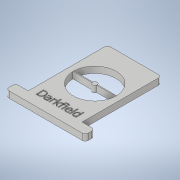
# Autodesk Inventor part: 00_Slider_Mask_Darkfield
Saved by Autodesk Inventor 2022 (Build 260153000, 153)
## iProperties
Created: 2021-10-22
Part Number: 00_Slider_Mask_Darkfield
Material: Generic
Document SubType Name: Modeling
Designer: diederichbenedict
Density: 1 g/cm^3
Appearance: Default
Author: diederichbenedict
Autodesk Inventor part; units mm, degrees
ref_plane "YZ Plane" through (0, 0, 0) normal (1, 0, 0) x (0, 1, 0)
ref_plane "XZ Plane" through (0, 0, 0) normal (0, 1, 0) x (-1, 0, 0)
ref_plane "XY Plane" through (0, 0, 0) normal (0, 0, 1) x (1, 0, 0)
sketch "Sketch1" plane through (0, 0, 0) normal (0, 1, 0) x (-1, 0, 0)
  line L0 (-17, 25) -> (17, 25)
  line L1 (17, 25) -> (17, -25)
  line L2 (17, -25) -> (-17, -25)
  line L3 (-17, -25) -> (-17, 25)
  line L4 (-17, 25) -> (17, -25) construction
  line L5 (17, 25) -> (-17, -25) construction
  line L6 (9, -17) -> (9, 17)
  line L7 (9, 17) -> (-9, 17)
  line L8 (-9, 17) -> (-9, -17)
  line L9 (-9, -17) -> (9, -17)
  line L10 (-25, 31) -> (25, 31)
  line L11 (25, 31) -> (25, 25)
  line L12 (25, 25) -> (-25, 25)
  line L13 (-25, 25) -> (-25, 31)
  line L14 (-25, 31) -> (25, 25) construction
  line L15 (25, 31) -> (-25, 25) construction
  point P0 (0, 0)
  point P1 (0, 28)
  point P2 (0, 25)
  dimension "d0" = 34
  dimension "d1" = 50
  dimension "d2" = 8
  dimension "d3" = 50
  dimension "d4" = 6
  constraints: 32 end point, 6 midpoint, 6 parallel, 3 perpendicular, 2 horizontal, 3 other
  measures "d0" distance of L1.end L2.end
  measures "d1" distance of L0.end L1.end
  measures "d2" distance between parallel lines of L1 L6
  measures "d3" distance of L11.end L12.end
  measures "d4" distance of L10.end L11.end
extrude "Extrusion1" add sketch "Sketch1" along normal blind 4 contours L12 L13 L10 L11 L0 | L0 L1 L2 L3 | L9 L8 L7 L6
sketch "Sketch2" plane through (0, 4, 0) normal (0, 1, 0) x (1, 0, 0)
  line L0 (25, -25) -> (17, -25)
  line L1 (17, -25) -> (17, 25)
  line L2 (17, 25) -> (-17, 25)
  line L3 (-17, 25) -> (-17, -25)
  line L4 (-17, -25) -> (-25, -25)
  line L5 (-25, -25) -> (-25, -31)
  line L6 (-25, -31) -> (25, -31)
  line L7 (25, -31) -> (25, -25)
  line L8 (13.5, 17) -> (-13.5, 17)
  line L9 (-13.5, 17) -> (-13.5, -17)
  line L10 (-13.5, -17) -> (13.5, -17)
  line L11 (13.5, -17) -> (13.5, 17)
  line L12 (13.5, 17) -> (-13.5, -17) construction
  line L13 (-13.5, 17) -> (13.5, -17) construction
  circle A0 centre (0, 0) radius 13.5
  circle A1 centre (0, 0) radius 1.5
  line L14 (-1.469694, 0.3) -> (-13.999729, 0.3)
  line L15 (-13.999729, 0.3) -> (-13.999729, -0.3)
  line L16 (-13.999729, -0.3) -> (-1.469694, -0.3)
  line L17 (-1.469694, -0.3) -> (-1.469694, 0.3)
  line L18 (1.469694, 0.3) -> (13.971759, 0.3)
  line L19 (13.971759, 0.3) -> (13.971759, -0.3)
  line L20 (13.971759, -0.3) -> (1.469694, -0.3)
  line L21 (1.469694, -0.3) -> (1.469694, 0.3)
  point P0 (13.496666, -0.3)
  point P1 (13.5, -0.3)
  point P2 (13.5, 0)
  point P3 (13.5, 0.3)
  point P4 (13.496666, 0.3)
  point P5 (1.469694, -0.3)
  point P6 (1.469694, -0.3)
  point P7 (-1.469694, -0.3)
  point P8 (-1.469694, -0.3)
  point P9 (-13.496666, -0.3)
  point P10 (-13.5, -0.3)
  point P11 (-13.5, 0)
  point P12 (-13.496666, 0.3)
  point P13 (-13.5, 0.3)
  dimension "d7" = 27
  dimension "d8" = 34
  dimension "d14" = 0.3
  dimension "d15" = 0.3
  dimension "d16" = 3
  constraints: 28 end point, 6 parallel, 3 horizontal, 3 perpendicular, 2 centre point, 2 coincident, 2 midpoint, 2 point on circle, 2 point on line
  measures "d7" distance of L10.end L9.end
  measures "d8" distance of L9.end L8.end
  measures "d14" distance from line of point (0, 0) L14
  measures "d15" distance from line of point (0, 0) L16
  measures "d16" diameter of A1
sketch "Sketch2 outline for Extrusion2" plane through (0, 4, 0) normal (0, 1, 0) x (1, 0, 0)
  line L0 (13.496666, -0.3) -> (13.5, -0.3)
  arc A0 (13.5, 0) -> (13.496666, -0.3) centre (0, 0) cw
  line L1 (13.5, -0.3) -> (13.5, 0)
  line L2 (13.5, 0.3) -> (13.496666, 0.3)
  line L3 (13.5, 0) -> (13.5, 0.3)
  arc A1 (13.496666, 0.3) -> (13.5, 0) centre (0, 0) cw
  line L4 (13.496666, -0.3) -> (1.469694, -0.3)
  arc A2 (-13.496666, -0.3) -> (13.496666, -0.3) centre (0, 0) ccw
  line L5 (-1.469694, -0.3) -> (-13.496666, -0.3)
  arc A3 (1.469694, -0.3) -> (-1.469694, -0.3) centre (0, 0) cw
  line L6 (-1.469694, -0.3) -> (-1.469694, 0.3)
  arc A4 (-1.469694, 0.3) -> (-1.469694, -0.3) centre (0, 0) ccw
  line L7 (-13.5, -0.3) -> (-13.496666, -0.3)
  line L8 (-13.5, 0) -> (-13.5, -0.3)
  arc A5 (-13.496666, -0.3) -> (-13.5, 0) centre (0, 0) cw
  line L9 (1.469694, 0.3) -> (1.469694, -0.3)
  arc A6 (1.469694, -0.3) -> (1.469694, 0.3) centre (0, 0) ccw
  line L10 (-13.496666, 0.3) -> (-13.5, 0.3)
  arc A7 (-13.5, 0) -> (-13.496666, 0.3) centre (0, 0) cw
  line L11 (-13.5, 0.3) -> (-13.5, 0)
  line L12 (1.469694, 0.3) -> (13.496666, 0.3)
  arc A8 (-1.469694, 0.3) -> (1.469694, 0.3) centre (0, 0) cw
  line L13 (-13.496666, 0.3) -> (-1.469694, 0.3)
  arc A9 (13.496666, 0.3) -> (-13.496666, 0.3) centre (0, 0) ccw
extrude "Extrusion2" cut sketch "Sketch2 outline for Extrusion2" against normal through all contours A0 L1 L0 | A2 L5 A3 L4 | A1 L2 L3 | L9 A6 | L7 L8 A5 | L12 A8 L13 A9 | A4 L6 | L11 L10 A7
sketch "Sketch3" plane through (0, 4, 0) normal (0, 1, 0) x (1, 0, 0)
  line L0 (-13.184715, -19.253856) -> (12.041103, -19.253856) construction
  line L1 (12.041103, -19.253856) -> (12.041103, -24.441026) construction
  line L2 (12.041103, -24.441026) -> (-13.184715, -24.441026) construction
  line L3 (-13.184715, -24.441026) -> (-13.184715, -19.253856) construction
  spline S0 degree 2 poles (-8.853526, -21.94014) (-8.853526, -22.60678) (-9.393939, -23.679716) (-9.84757, -23.979506) knots 0 0 0 1 2 2 2
  spline S1 degree 2 poles (-9.84757, -23.979506) (-10.218364, -24.212239) (-10.979674, -24.370023) (-11.571367, -24.370023) knots 0 0 0 1 2 2 2
  line L4 (-11.571367, -24.370023) -> (-12.691638, -24.370023)
  line L5 (-12.691638, -24.370023) -> (-12.691638, -19.502367)
  line L6 (-12.691638, -19.502367) -> (-11.583201, -19.502367)
  spline S2 degree 2 poles (-11.583201, -19.502367) (-10.896837, -19.502367) (-10.115804, -19.707487) (-9.83968, -19.88894) knots 0 0 0 1 2 2 2
  spline S3 degree 2 poles (-9.83968, -19.88894) (-9.370271, -20.200564) (-8.853526, -21.230109) (-8.853526, -21.94014) knots 0 0 0 1 2 2 2
  spline S4 degree 2 poles (-9.528056, -21.932251) (-9.528056, -21.372115) (-9.89885, -20.579248) (-10.265699, -20.354404) knots 0 0 0 1 2 2 2
  spline S5 degree 2 poles (-10.265699, -20.354404) (-10.526044, -20.200564) (-11.113791, -20.062503) (-11.551644, -20.062503) knots 0 0 0 1 2 2 2
  line L7 (-11.551644, -20.062503) -> (-12.044721, -20.062503)
  line L8 (-12.044721, -20.062503) -> (-12.044721, -23.809888)
  line L9 (-12.044721, -23.809888) -> (-11.551644, -23.809888)
  spline S6 degree 2 poles (-11.551644, -23.809888) (-11.121681, -23.809888) (-10.470819, -23.671826) (-10.20653, -23.486429) knots 0 0 0 1 2 2 2
  spline S7 degree 2 poles (-10.20653, -23.486429) (-9.867293, -23.257642) (-9.528056, -22.500275) (-9.528056, -21.932251) knots 0 0 0 1 2 2 2
  spline S8 degree 2 poles (-6.163298, -23.983451) (-6.238246, -24.038676) (-6.490702, -24.235906) (-6.60904, -24.295076) knots 0 0 0 1 2 2 2
  spline S9 degree 2 poles (-6.60904, -24.295076) (-6.770769, -24.381857) (-7.074505, -24.472583) (-7.350628, -24.472583) knots 0 0 0 1 2 2 2
  spline S10 degree 2 poles (-7.350628, -24.472583) (-7.575471, -24.472583) (-7.981766, -24.302965) (-8.135606, -24.149125) knots 0 0 0 1 2 2 2
  spline S11 degree 2 poles (-8.135606, -24.149125) (-8.281557, -23.999229) (-8.459065, -23.557432) (-8.459065, -23.312866) knots 0 0 0 1 2 2 2
  spline S12 degree 2 poles (-8.459065, -23.312866) (-8.459065, -22.934183) (-8.139551, -22.397715) (-7.792425, -22.243875) knots 0 0 0 1 2 2 2
  spline S13 degree 2 poles (-7.792425, -22.243875) (-7.484745, -22.101869) (-6.648486, -21.995365) (-6.163298, -21.967752) knots 0 0 0 1 2 2 2
  line L10 (-6.163298, -21.967752) -> (-6.163298, -21.849414)
  spline S14 degree 2 poles (-6.163298, -21.849414) (-6.163298, -21.636405) (-6.293471, -21.372115) (-6.411809, -21.297168) knots 0 0 0 1 2 2 2
  spline S15 degree 2 poles (-6.411809, -21.297168) (-6.530148, -21.22222) (-6.869385, -21.174885) (-7.050837, -21.174885) knots 0 0 0 1 2 2 2
  spline S16 degree 2 poles (-7.050837, -21.174885) (-7.263846, -21.174885) (-7.83976, -21.301112) (-8.127717, -21.423395) knots 0 0 0 1 2 2 2
  line L11 (-8.127717, -21.423395) -> (-8.163219, -21.423395)
  line L12 (-8.163219, -21.423395) -> (-8.163219, -20.796201)
  spline S17 degree 2 poles (-8.163219, -20.796201) (-7.9936, -20.748866) (-7.358517, -20.630528) (-7.046892, -20.630528) knots 0 0 0 1 2 2 2
  spline S18 degree 2 poles (-7.046892, -20.630528) (-6.668209, -20.630528) (-6.151465, -20.748866) (-5.946345, -20.902706) knots 0 0 0 1 2 2 2
  spline S19 degree 2 poles (-5.946345, -20.902706) (-5.745169, -21.052601) (-5.547938, -21.5299) (-5.547938, -21.873082) knots 0 0 0 1 2 2 2
  line L13 (-5.547938, -21.873082) -> (-5.547938, -24.370023)
  line L14 (-5.547938, -24.370023) -> (-6.163298, -24.370023)
  line L15 (-6.163298, -24.370023) -> (-6.163298, -23.983451)
  line L16 (-6.163298, -23.470651) -> (-6.163298, -22.456885)
  spline S20 degree 2 poles (-6.163298, -22.456885) (-6.384197, -22.476608) (-7.050837, -22.543666) (-7.259902, -22.60678) knots 0 0 0 1 2 2 2
  spline S21 degree 2 poles (-7.259902, -22.60678) (-7.504468, -22.681728) (-7.823982, -22.993352) (-7.823982, -23.269476) knots 0 0 0 1 2 2 2
  spline S22 degree 2 poles (-7.823982, -23.269476) (-7.823982, -23.585045) (-7.468966, -23.904559) (-7.129729, -23.904559) knots 0 0 0 1 2 2 2
  spline S23 degree 2 poles (-7.129729, -23.904559) (-6.841772, -23.904559) (-6.368418, -23.656048) (-6.163298, -23.470651) knots 0 0 0 1 2 2 2
  line L17 (-2.747261, -21.37606) -> (-2.778818, -21.37606)
  spline S24 degree 2 poles (-2.778818, -21.37606) (-2.849821, -21.356337) (-3.003661, -21.348448) (-3.110166, -21.348448) knots 0 0 0 1 2 2 2
  spline S25 degree 2 poles (-3.110166, -21.348448) (-3.358677, -21.348448) (-3.847809, -21.565401) (-4.068707, -21.778411) knots 0 0 0 1 2 2 2
  line L18 (-4.068707, -21.778411) -> (-4.068707, -24.370023)
  line L19 (-4.068707, -24.370023) -> (-4.684068, -24.370023)
  line L20 (-4.684068, -24.370023) -> (-4.684068, -20.717309)
  line L21 (-4.684068, -20.717309) -> (-4.068707, -20.717309)
  line L22 (-4.068707, -20.717309) -> (-4.068707, -21.261666)
  spline S26 degree 2 poles (-4.068707, -21.261666) (-3.733415, -20.961875) (-3.232449, -20.717309) (-2.995772, -20.717309) knots 0 0 0 1 2 2 2
  spline S27 degree 2 poles (-2.995772, -20.717309) (-2.901101, -20.717309) (-2.80643, -20.725198) (-2.747261, -20.737032) knots 0 0 0 1 2 2 2
  line L23 (-2.747261, -20.737032) -> (-2.747261, -21.37606)
  line L24 (0.755558, -24.370023) -> (-0.053089, -24.370023)
  line L25 (-0.053089, -24.370023) -> (-1.410036, -22.60678)
  line L26 (-1.410036, -22.60678) -> (-1.654603, -22.843457)
  line L27 (-1.654603, -22.843457) -> (-1.654603, -24.370023)
  line L28 (-1.654603, -24.370023) -> (-2.269963, -24.370023)
  line L29 (-2.269963, -24.370023) -> (-2.269963, -19.285414)
  line L30 (-2.269963, -19.285414) -> (-1.654603, -19.285414)
  line L31 (-1.654603, -19.285414) -> (-1.654603, -22.259654)
  line L32 (-1.654603, -22.259654) -> (-0.210873, -20.717309)
  line L33 (-0.210873, -20.717309) -> (0.554382, -20.717309)
  line L34 (0.554382, -20.717309) -> (-0.944572, -22.243875)
  line L35 (-0.944572, -22.243875) -> (0.755558, -24.370023)
  line L36 (2.984266, -19.877106) -> (2.952709, -19.877106)
  spline S28 degree 2 poles (2.952709, -19.877106) (2.869872, -19.845549) (2.562192, -19.790324) (2.439909, -19.790324) knots 0 0 0 1 2 2 2
  spline S29 degree 2 poles (2.439909, -19.790324) (2.053336, -19.790324) (1.721989, -20.137451) (1.721989, -20.595026) knots 0 0 0 1 2 2 2
  line L37 (1.721989, -20.595026) -> (1.721989, -20.717309)
  line L38 (1.721989, -20.717309) -> (2.739699, -20.717309)
  line L39 (2.739699, -20.717309) -> (2.739699, -21.226165)
  line L40 (2.739699, -21.226165) -> (1.741712, -21.226165)
  line L41 (1.741712, -21.226165) -> (1.741712, -24.370023)
  line L42 (1.741712, -24.370023) -> (1.126352, -24.370023)
  line L43 (1.126352, -24.370023) -> (1.126352, -21.226165)
  line L44 (1.126352, -21.226165) -> (0.712167, -21.226165)
  line L45 (0.712167, -21.226165) -> (0.712167, -20.717309)
  line L46 (0.712167, -20.717309) -> (1.126352, -20.717309)
  line L47 (1.126352, -20.717309) -> (1.126352, -20.595026)
  spline S30 degree 2 poles (1.126352, -20.595026) (1.126352, -19.94022) (1.761435, -19.253857) (2.353127, -19.253857) knots 0 0 0 1 2 2 2
  spline S31 degree 2 poles (2.353127, -19.253857) (2.522746, -19.253857) (2.850149, -19.289358) (2.984266, -19.313026) knots 0 0 0 1 2 2 2
  line L48 (2.984266, -19.313026) -> (2.984266, -19.877106)
  line L49 (3.820524, -24.370023) -> (3.205164, -24.370023)
  line L50 (3.205164, -24.370023) -> (3.205164, -20.717309)
  line L51 (3.205164, -20.717309) -> (3.820524, -20.717309)
  line L52 (3.820524, -20.717309) -> (3.820524, -24.370023)
  line L53 (3.863915, -20.109838) -> (3.165718, -20.109838)
  line L54 (3.165718, -20.109838) -> (3.165718, -19.47081)
  line L55 (3.165718, -19.47081) -> (3.863915, -19.47081)
  line L56 (3.863915, -19.47081) -> (3.863915, -20.109838)
  spline S32 degree 2 poles (6.309577, -24.45286) (5.433872, -24.45286) (4.471386, -23.470651) (4.471386, -22.563389) knots 0 0 0 1 2 2 2
  spline S33 degree 2 poles (4.471386, -22.563389) (4.471386, -21.671906) (5.40626, -20.614749) (6.159681, -20.614749) knots 0 0 0 1 2 2 2
  spline S34 degree 2 poles (6.159681, -20.614749) (6.498918, -20.614749) (7.023552, -20.81198) (7.216838, -21.021045) knots 0 0 0 1 2 2 2
  spline S35 degree 2 poles (7.216838, -21.021045) (7.414069, -21.230109) (7.623134, -21.833635) (7.623134, -22.271488) knots 0 0 0 1 2 2 2
  line L57 (7.623134, -22.271488) -> (7.623134, -22.60678)
  line L58 (7.623134, -22.60678) -> (5.094635, -22.60678)
  spline S36 degree 2 poles (5.094635, -22.60678) (5.094635, -23.241863) (5.733663, -23.916393) (6.301688, -23.916393) knots 0 0 0 1 2 2 2
  spline S37 degree 2 poles (6.301688, -23.916393) (6.502863, -23.916393) (6.89338, -23.825666) (7.051165, -23.754663) knots 0 0 0 1 2 2 2
  spline S38 degree 2 poles (7.051165, -23.754663) (7.216838, -23.675771) (7.445626, -23.537709) (7.520574, -23.474596) knots 0 0 0 1 2 2 2
  line L59 (7.520574, -23.474596) -> (7.556075, -23.474596)
  line L60 (7.556075, -23.474596) -> (7.556075, -24.14518)
  spline S39 degree 2 poles (7.556075, -24.14518) (7.449571, -24.188571) (7.126112, -24.314799) (6.999885, -24.3503) knots 0 0 0 1 2 2 2
  spline S40 degree 2 poles (6.999885, -24.3503) (6.822377, -24.40158) (6.530475, -24.45286) (6.309577, -24.45286) knots 0 0 0 1 2 2 2
  spline S41 degree 2 poles (7.023552, -22.137371) (7.015663, -21.88886) (6.913103, -21.525955) (6.814488, -21.403672) knots 0 0 0 1 2 2 2
  spline S42 degree 2 poles (6.814488, -21.403672) (6.707983, -21.265611) (6.372691, -21.11966) (6.12418, -21.11966) knots 0 0 0 1 2 2 2
  spline S43 degree 2 poles (6.12418, -21.11966) (5.879614, -21.11966) (5.536432, -21.265611) (5.394426, -21.407617) knots 0 0 0 1 2 2 2
  spline S44 degree 2 poles (5.394426, -21.407617) (5.256364, -21.553568) (5.114358, -21.904638) (5.094635, -22.137371) knots 0 0 0 1 2 2 2
  line L61 (5.094635, -22.137371) -> (7.023552, -22.137371)
  line L62 (8.873577, -24.370023) -> (8.258217, -24.370023)
  line L63 (8.258217, -24.370023) -> (8.258217, -19.285414)
  line L64 (8.258217, -19.285414) -> (8.873577, -19.285414)
  line L65 (8.873577, -19.285414) -> (8.873577, -24.370023)
  line L66 (12.585461, -24.370023) -> (11.970101, -24.370023)
  line L67 (11.970101, -24.370023) -> (11.970101, -23.999229)
  spline S45 degree 2 poles (11.970101, -23.999229) (11.828094, -24.117568) (11.61903, -24.275353) (11.477024, -24.342411) knots 0 0 0 1 2 2 2
  spline S46 degree 2 poles (11.477024, -24.342411) (11.346851, -24.405525) (11.066783, -24.472583) (10.881387, -24.472583) knots 0 0 0 1 2 2 2
  spline S47 degree 2 poles (10.881387, -24.472583) (10.581596, -24.472583) (10.076685, -24.224073) (9.899177, -23.983451) knots 0 0 0 1 2 2 2
  spline S48 degree 2 poles (9.899177, -23.983451) (9.721669, -23.742829) (9.524439, -23.032799) (9.524439, -22.571279) knots 0 0 0 1 2 2 2
  spline S49 degree 2 poles (9.524439, -22.571279) (9.524439, -22.090035) (9.772949, -21.387894) (9.989903, -21.123605) knots 0 0 0 1 2 2 2
  spline S50 degree 2 poles (9.989903, -21.123605) (10.191079, -20.886928) (10.755159, -20.614749) (11.066783, -20.614749) knots 0 0 0 1 2 2 2
  spline S51 degree 2 poles (11.066783, -20.614749) (11.338962, -20.614749) (11.745257, -20.737032) (11.970101, -20.86326) knots 0 0 0 1 2 2 2
  line L68 (11.970101, -20.86326) -> (11.970101, -19.285414)
  line L69 (11.970101, -19.285414) -> (12.585461, -19.285414)
  line L70 (12.585461, -19.285414) -> (12.585461, -24.370023)
  line L71 (11.970101, -23.482485) -> (11.970101, -21.372115)
  spline S52 degree 2 poles (11.970101, -21.372115) (11.741313, -21.261666) (11.378408, -21.178829) (11.169344, -21.178829) knots 0 0 0 1 2 2 2
  spline S53 degree 2 poles (11.169344, -21.178829) (10.69599, -21.178829) (10.159522, -21.88886) (10.159522, -22.559445) knots 0 0 0 1 2 2 2
  spline S54 degree 2 poles (10.159522, -22.559445) (10.159522, -23.206362) (10.569762, -23.88878) (11.023393, -23.88878) knots 0 0 0 1 2 2 2
  spline S55 degree 2 poles (11.023393, -23.88878) (11.264014, -23.88878) (11.753147, -23.667882) (11.970101, -23.482485) knots 0 0 0 1 2 2 2
  point P0 (0, 0)
  constraints: 2 other
extrude "Extrusion3" cut sketch "Sketch3" against normal blind 1
fillet "Fillet1" radius 2 6 edges at (25, 2, 31) (25, 2, 25) (-25, 2, 31) (-25, 2, 25) (-17, 2, -25) (17, 2, -25)
body "Solid1"
